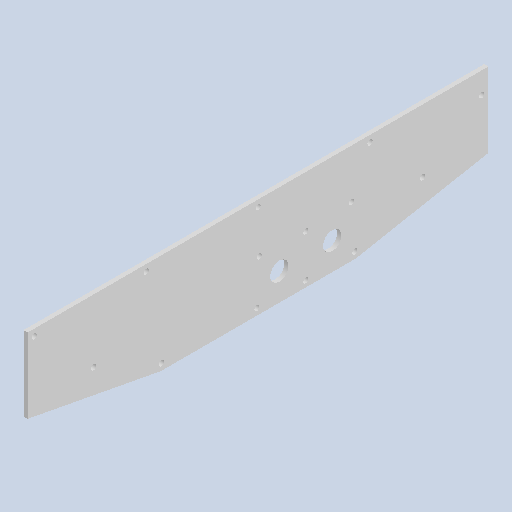
# Autodesk Inventor part: InsideChassiPlate3.0
Saved by Autodesk Inventor 2023 (Build 270158000, 158)
## iProperties
Created: 2022-09-18
Part Number: InsideChassiPlate3.0
Material: Generic
Document SubType Name: Modeling
Designer: deli
Density: 1 g/cm^3
Appearance: Default
Mass: 76.7316 g
Surface Area: 518.075 cm^2
Volume: 76.7316 cm^3
Author: deli
Autodesk Inventor part; units mm, degrees
ref_plane "YZ Plane" through (0, 0, 0) normal (1, 0, 0) x (0, 1, 0)
ref_plane "XZ Plane" through (0, 0, 0) normal (0, 1, 0) x (-1, 0, 0)
ref_plane "XY Plane" through (0, 0, 0) normal (0, 0, 1) x (1, 0, 0)
sketch "Sketch1" plane through (0, 0, 0) normal (1, 0, 0) x (0, 1, 0)
  line L0 (161.267, 41.7418) -> (161.267, -105.149) projected
  arc A0 (161.267, -105.149) -> (161.3544, -106.0799) centre (166.267, -105.149) ccw projected
  line L1 (161.3544, -106.0799) -> (180.4208, -206.7036) projected
  line L2 (180.4208, -206.7036) -> (253.267, -206.7036) projected
  line L3 (253.267, -206.7036) -> (253.267, 143.2964) projected
  line L4 (253.267, 143.2964) -> (180.4208, 143.2964) projected
  line L5 (180.4208, 143.2964) -> (161.3544, 42.6727) projected
  arc A1 (161.3544, 42.6727) -> (161.267, 41.7418) centre (166.267, 41.7418) ccw projected
  circle A2 centre (232.267, 53.2964) radius 2 projected
  circle A3 centre (232.267, -116.7036) radius 2 projected
  circle A4 centre (220.8897, -201.7036) radius 2 projected
  circle A5 centre (200.186, -102.5532) radius 2 projected
  circle A6 centre (166.267, -30.806) radius 2 projected
  circle A7 centre (165.883, -67.9775) radius 2 projected
  circle A8 centre (198.1509, -67.9775) radius 2 projected
  circle A9 centre (182.017, -88.0464) radius 7 projected
  circle A10 centre (182.017, -47.9087) radius 7 projected
  circle A11 centre (189.267, -156.7036) radius 2 projected
  circle A12 centre (189.267, 93.2964) radius 2 projected
  circle A13 centre (232.267, 138.2964) radius 2 projected
  circle A14 centre (199.4689, -32.5466) radius 2 projected
  circle A15 centre (232.267, -31.7036) radius 2 projected
  circle A16 centre (166.267, 41.7418) radius 2 projected
  circle A17 centre (166.267, -105.149) radius 2 projected
  line L6 (237.267, 143.2964) -> (237.267, -206.7036)
  point P0 (0, 0)
  dimension "d6" = 16
  constraints: 2 end point, 2 point on line, 1 vertical
  measures "d6" distance between parallel lines of L3 L6
extrude "Extrusion1" add sketch "Sketch1" along normal blind 3.175 contours A1 L5 L4 L6 L2 L1 A0 L0
body "Solid1"
